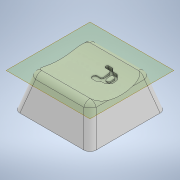
# Autodesk Inventor part: KeycapA
Saved by Autodesk Inventor 2022 (Build 260153000, 153)
## iProperties
Created: 2022-03-01
Part Number: KeycapA
Material: Generic
Document SubType Name: Modeling
Designer: Nathan Griffith
Density: 1 g/cm^3
Appearance: Default
Author: Nathan Griffith
Autodesk Inventor part; units mm, degrees
ref_plane "YZ Plane" through (0, 0, 0) normal (1, 0, 0) x (0, 1, 0)
ref_plane "XZ Plane" through (0, 0, 0) normal (0, 1, 0) x (-1, 0, 0)
ref_plane "XY Plane" through (0, 0, 0) normal (0, 0, 1) x (1, 0, 0)
sketch "Sketch1" plane through (0, 0, 0) normal (0, 1, 0) x (-1, 0, 0)
  line L0 (0, 0) -> (18, 0)
  line L1 (18, 0) -> (18, 18)
  line L2 (18, 18) -> (0, 18)
  line L3 (0, 18) -> (0, 0)
  dimension "d0" = 18
  dimension "d1" = 18
  constraints: 8 end point, 2 parallel, 1 horizontal, 1 perpendicular
  measures "d0" distance of L2.end L1.end
  measures "d1" distance of L1.end L0.end
extrude "Extrusion1" add sketch "Sketch1" along normal blind 8 draft -15
fillet "Fillet1" radius 1.5 8 edges at (-1.0718, 4, 16.9282) (-9, 8, 15.8564) (-2.1436, 8, 9) (-9, 8, 2.1436) (-1.0718, 4, 1.0718) (-16.9282, 4, 1.0718) (-16.9282, 4, 16.9282) (-15.8564, 8, 9)
ref_plane "Work Plane1" through (-9, 33.5885, 16.5511) normal (1, 0, 0) x (0, 0, -1)
sketch "Sketch2" plane through (-9, 33.5885, 16.5511) normal (1, 0, 0) x (0, 0, -1)
  line L0 (13.2565, -25.5885) -> (1.8457, -25.5885) projected
  arc A0 (14.7054, -26.7002) -> (13.2565, -25.5885) centre (13.2565, -27.0885) ccw projected
  arc A1 (1.8457, -25.5885) -> (13.2565, -25.5885) centre (7.5511, -15.0316) ccw
  point P0 (16.5511, -33.5885)
  point P1 (13.2565, -25.5885)
  dimension "d5" = 12
  constraints: 3 point on circle, 1 centre point
  measures "d5" radius of A1
extrude "Extrusion2" cut sketch "Sketch2" along normal through all both and the other way through all
sketch "Sketch3" plane through (0, 0, 0) normal (0, -1, 0) x (1, 0, 0)
  line L0 (-16.5511, 18) -> (-1.4489, 18) construction
  line L1 (-9, 18) -> (-9, 0) construction
  line L2 (-1.4489, 0) -> (-16.5511, 0) construction
  line L3 (-18, 1.4489) -> (-18, 16.5511) construction
  line L4 (-18, 9) -> (0, 9) construction
  line L5 (-1, 1) -> (-17, 1)
  line L6 (-17, 1) -> (-17, 17)
  line L7 (-17, 17) -> (-1, 17)
  line L8 (-1, 17) -> (-1, 1)
  line L9 (-1, 1) -> (-17, 17) construction
  line L10 (-17, 1) -> (-1, 17) construction
  point P0 (0, 0)
  point P1 (-9, 9)
  point P2 (-9, 9)
  dimension "d8" = 16
  dimension "d9" = 16
  constraints: 16 end point, 8 midpoint, 2 horizontal, 2 parallel, 1 perpendicular
  measures "d8" distance of L6.end L7.end
  measures "d9" distance of L7.end L5.start
extrude "Extrusion3" cut sketch "Sketch3" against normal blind 4.5 draft -15
sketch "Sketch4" plane through (0, 4.5, 0) normal (0, -1, 0) x (1, 0, 0)
  line L0 (-15.7942, 15.7942) -> (-15.7942, 2.2058) construction
  line L1 (-15.7942, 9) -> (-2.2058, 9) construction
  line L2 (-2.2058, 2.2058) -> (-2.2058, 15.7942) construction
  line L3 (-2.2058, 15.7942) -> (-15.7942, 15.7942) construction
  line L4 (-9, 15.7942) -> (-9, 2.2058) construction
  line L5 (-15.7942, 2.2058) -> (-2.2058, 2.2058) construction
  circle A0 centre (-9, 9) radius 2.775
  point P0 (0, 0)
  dimension "d12" = 5.55
  constraints: 5 midpoint, 4 end point, 1 centre point
  measures "d12" diameter of A0
extrude "Extrusion4" add sketch "Sketch4" along normal blind 4
sketch "Sketch5" plane through (-9, 0.5, 9) normal (0, -1, 0) x (1, 0, 0)
  line L0 (0.6, 2.075) -> (-0.6, 2.075)
  line L1 (-0.6, -2.075) -> (0.6, -2.075)
  line L2 (-0.6, 2.075) -> (0.6, -2.075) construction
  line L3 (-2.075, 0.6) -> (-2.075, -0.6)
  line L4 (2.075, -0.6) -> (2.075, 0.6)
  line L5 (2.075, 0.6) -> (-2.075, -0.6) construction
  line L6 (-2.075, 0.6) -> (2.075, -0.6) construction
  line L7 (-6.7942, 6.7942) -> (-6.7942, -6.7942) construction
  line L8 (-6.7942, 0) -> (6.7942, 0) construction
  line L9 (6.7942, -6.7942) -> (6.7942, 6.7942) construction
  line L10 (-6.7942, -6.7942) -> (6.7942, -6.7942) construction
  line L11 (0, -6.7942) -> (0, 6.7942) construction
  arc A0 (0.9, -0.6) -> (0.6, -0.9) centre (0.9, -0.9) ccw
  arc A1 (-0.6, -0.9) -> (-0.9, -0.6) centre (-0.9, -0.9) ccw
  arc A2 (0.6, 0.9) -> (0.9, 0.6) centre (0.9, 0.9) ccw
  arc A3 (-0.9, 0.6) -> (-0.6, 0.9) centre (-0.9, 0.9) ccw
  line L12 (-0.6, 2.075) -> (-0.6, 0.9)
  line L13 (-0.6, -0.9) -> (-0.6, -2.075)
  line L14 (-2.075, -0.6) -> (-0.9, -0.6)
  line L15 (-0.9, 0.6) -> (-2.075, 0.6)
  line L16 (0.6, 2.075) -> (0.1735, 0.6) construction
  line L17 (0, 0) -> (-0.6, -2.075) construction
  line L18 (2.075, 0.6) -> (0.9, 0.6)
  line L19 (0.9, -0.6) -> (2.075, -0.6)
  line L20 (0.6, -2.075) -> (0.6, -0.9)
  line L21 (0.6, 0.9) -> (0.6, 2.075)
  point P0 (9, -9)
  dimension "d15" = 1.2
  dimension "d16" = 4.15
  dimension "d17" = 4.15
  dimension "d18" = 1.2
  dimension "d19" = 0.3
  constraints: 38 end point, 10 parallel, 9 midpoint, 9 symmetric about line, 8 point on circle, 4 centre point, 4 perpendicular, 4 tangent, 3 horizontal, 1 vertical, 3 other
  measures "d15" distance of L1.end L1.start
  measures "d16" distance of L1.start L0.end
  measures "d17" distance of L4.start L3.end
  measures "d18" distance of L3.end L3.start
  measures "d19" radius of A0
extrude "Extrusion5" cut sketch "Sketch5" against normal blind 4
ref_plane "Work Plane2" through (-13.5, 8, 3.2946) normal (0, -1, 0) x (1, 0, 0)
sketch "Sketch6" plane through (-13.5, 8, 3.2946) normal (0, -1, 0) x (1, 0, 0)
  ellipse E0 centre (8.5277, 5.7054) end of major axis (8.5277, 17.7054) minor radius 3.2154 (11.6543, 2.9051) -> (11.6543, 8.5058) ccw construction
  line L0 (11.6543, 2.9051) -> (11.6543, 8.5058) construction
  ellipse E1 centre (0.4723, 5.7054) end of major axis (0.4723, -6.2946) minor radius 3.2154 (-2.6543, 8.5058) -> (-2.6543, 2.9051) ccw construction
  line L1 (-2.6543, 2.9051) -> (-2.6543, 8.5058) construction
  line L2 (11.6543, 5.7054) -> (4.4996, 5.8101) construction
  line L3 (-1.2054, 0) -> (10.2054, 0) construction
  line L4 (4.5, 0) -> (4.4996, 5.8101) construction
  line L5 (10.2054, 11.4108) -> (-1.2054, 11.4108) construction
  line L6 (4.4996, 5.8101) -> (4.5, 11.4108) construction
  line L7 (4.4996, 5.8101) -> (-2.6543, 5.7054) construction
  line L8 (4.4998, 2.9051) -> (11.6543, 2.9051) construction
  line L9 (8.077, 5.7578) -> (8.077, 0) construction
  spline S0 degree 2 poles (6.0608, 5.6859) (6.0841, 5.6626) (6.1954, 5.5565) (6.3249, 5.4322) (6.4388, 5.3261) (6.4621, 5.3028) knots 0 0 0 1 2 3 4 4 4
  spline S1 degree 2 poles (6.4621, 5.3028) (6.4984, 5.2717) (6.6511, 5.2018) (6.6874, 5.2018) knots 0 0 0 1 2 2 2
  line L10 (6.6874, 5.2018) -> (7.6039, 5.2019)
  line L11 (7.6039, 5.2019) -> (7.7385, 5.1242)
  line L12 (7.7385, 5.1242) -> (8.4298, 4.433)
  line L13 (8.4298, 4.433) -> (8.4945, 4.2984)
  line L14 (8.4945, 4.2984) -> (8.5179, 3.3819)
  spline S2 degree 2 poles (8.5179, 3.3819) (8.5179, 3.3275) (8.4713, 3.1515) (8.4299, 3.1152) knots 0 0 0 1 2 2 2
  line L15 (8.4299, 3.1152) -> (7.7387, 2.4187)
  spline S3 degree 2 poles (7.7387, 2.4187) (7.7206, 2.4058) (7.6507, 2.3695) (7.5678, 2.3411) (7.4901, 2.3178) (7.4668, 2.3178) knots 0 0 0 1 2 3 4 4 4
  line L16 (7.4668, 2.3178) -> (6.5969, 2.3177)
  line L17 (6.5969, 2.3177) -> (6.4623, 2.24)
  line L18 (6.4623, 2.24) -> (6.061, 1.862)
  spline S4 degree 2 poles (6.061, 1.862) (6.0119, 1.8206) (5.8539, 1.774) (5.7944, 1.774) knots 0 0 0 1 2 2 2
  line L19 (5.7944, 1.774) -> (4.984, 1.7739)
  spline S5 degree 2 poles (4.984, 1.7739) (4.8494, 1.7739) (4.606, 1.9551) (4.606, 2.0975) knots 0 0 0 1 2 2 2
  spline S6 degree 2 poles (4.606, 2.0975) (4.606, 2.1467) (4.6526, 2.2528) (4.7303, 2.3461) (4.8312, 2.4108) (4.8778, 2.4108) knots 0 0 0 1 2 3 4 4 4
  line L20 (4.8778, 2.4108) -> (5.7943, 2.4108)
  spline S7 degree 2 poles (5.7943, 2.4108) (5.8409, 2.4109) (5.9704, 2.4704) (6.0895, 2.5584) (6.1723, 2.6775) (6.1723, 2.7319) knots 0 0 0 1 2 3 4 4 4
  line L21 (6.1723, 2.7319) -> (6.1722, 4.2568)
  spline S8 degree 2 poles (6.1722, 4.2568) (6.1722, 4.2905) (6.1075, 4.3915) (6.0194, 4.4924) (5.9185, 4.5571) (5.8822, 4.5571) knots 0 0 0 1 2 3 4 4 4
  line L22 (5.8822, 4.5571) -> (4.9838, 4.5571)
  spline S9 degree 2 poles (4.9838, 4.5571) (4.9657, 4.5571) (4.8958, 4.5804) (4.8181, 4.6166) (4.7534, 4.6529) (4.7431, 4.658) knots 0 0 0 1 2 3 4 4 4
  spline S10 degree 2 poles (4.7431, 4.658) (4.6058, 4.759) (4.5178, 5.0127) (4.5178, 5.1706) knots 0 0 0 1 2 2 2
  spline S11 degree 2 poles (4.5178, 5.1706) (4.5178, 5.3312) (4.6058, 5.5849) (4.743, 5.6859) knots 0 0 0 1 2 2 2
  spline S12 degree 2 poles (4.743, 5.6859) (4.7585, 5.6988) (4.8673, 5.7506) (4.8776, 5.7506) knots 0 0 0 1 2 2 2
  line L23 (4.8776, 5.7506) -> (5.9236, 5.7507)
  line L24 (5.9236, 5.7507) -> (6.0608, 5.6859)
  spline S13 degree 2 poles (7.3555, 2.9779) (7.4202, 2.9779) (7.5911, 3.0142) (7.7438, 3.0867) (7.85, 3.2032) (7.8499, 3.2912) knots 0 0 0 1 2 3 4 4 4
  line L25 (7.8499, 3.2912) -> (7.8499, 4.2569)
  spline S14 degree 2 poles (7.8499, 4.2569) (7.8499, 4.2906) (7.7851, 4.3916) (7.6971, 4.4796) (7.5961, 4.5443) (7.5547, 4.5443) knots 0 0 0 1 2 3 4 4 4
  line L26 (7.5547, 4.5443) -> (7.1534, 4.5443)
  spline S15 degree 2 poles (7.1534, 4.5443) (7.0887, 4.5443) (6.9774, 4.4614) (6.8945, 4.3397) (6.8402, 4.1973) (6.8402, 4.143) knots 0 0 0 1 2 3 4 4 4
  line L27 (6.8402, 4.143) -> (6.8402, 3.3818)
  spline S16 degree 2 poles (6.8402, 3.3818) (6.8402, 3.2808) (6.936, 3.1281) (7.0888, 3.0271) (7.2726, 2.9779) (7.3555, 2.9779) knots 0 0 0 1 2 3 4 4 4
  point P0 (13.5, -3.2946)
  constraints: 16 end point, 6 midpoint, 3 vertical, 1 horizontal, 1 point on line, 3 other
extrude "Extrusion6" cut sketch "Sketch6" along normal blind 1.6
body "Solid1"
